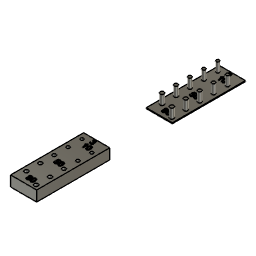
03 mm 3D Holes and Pins Kit v2 (Autodesk Fusion 360 design; units mm, degrees)
Autodesk Fusion 360 part; units mm, degrees
sketch "Schizzo1" plane through (0, 0, 0) normal (0, 0, 1) x (1, 0, 0)
  circle A0 centre (-272.0657, 86.4576) radius 1.5
  circle A1 centre (-256.0657, 66.4576) radius 1.65
  line L0 (-276.5657, 92.4576) -> (-251.5657, 92.4576)
  line L1 (-276.5657, 59.7909) -> (-251.5657, 59.7909) construction
  circle A2 centre (-272.0657, 73.1243) radius 1.6
  line L2 (-276.5657, 33.1243) -> (-251.5657, 33.1243) construction
  line L3 (-276.5657, 79.7909) -> (-251.5657, 79.7909) construction
  line L4 (-251.5657, 22.4576) -> (-276.5657, 22.4576)
  line L5 (-276.5657, 26.4576) -> (-251.5657, 26.4576) construction
  circle A3 centre (-256.0657, 39.7909) radius 1.85
  circle A4 centre (-272.0657, 33.1243) radius 1.9
  line L6 (-276.5657, 53.1243) -> (-251.5657, 53.1243) construction
  line L7 (-276.5657, 46.4576) -> (-251.5657, 46.4576) construction
  line L8 (-276.5657, 39.7909) -> (-251.5657, 39.7909) construction
  circle A5 centre (-256.0657, 26.4576) radius 1.95
  circle A6 centre (-272.0657, 46.4576) radius 1.8
  line L9 (-251.5657, 92.4576) -> (-251.5657, 22.4576)
  line L10 (-276.5657, 66.4576) -> (-251.5657, 66.4576) construction
  circle A7 centre (-256.0657, 53.1243) radius 1.75
  line L11 (-256.0657, 92.4576) -> (-256.0657, 22.4576) construction
  line L12 (-276.5657, 73.1243) -> (-251.5657, 73.1243) construction
  circle A8 centre (-272.0657, 59.7909) radius 1.7
  circle A9 centre (-256.0657, 79.7909) radius 1.55
  line L13 (-272.0657, 92.4576) -> (-272.0657, 22.4576) construction
  line L14 (-276.5657, 86.4576) -> (-251.5657, 86.4576) construction
  line L15 (-276.5657, 22.4576) -> (-276.5657, 92.4576)
  line L16 (-264.0657, 92.4576) -> (-264.0657, 22.4576) construction
  line L17 (-276.5657, -43.5424) -> (-251.5657, -43.5424) construction
  line L18 (-256.0657, -37.5424) -> (-256.0657, -107.5424) construction
  line L19 (-276.5657, -103.5424) -> (-251.5657, -103.5424) construction
  circle A10 centre (-256.0657, -103.5424) radius 1.95
  line L20 (-276.5657, -50.2091) -> (-251.5657, -50.2091) construction
  line L21 (-276.5657, -76.8757) -> (-251.5657, -76.8757) construction
  circle A11 centre (-272.0657, -56.8757) radius 1.6
  line L22 (-276.5657, -37.5424) -> (-251.5657, -37.5424)
  circle A12 centre (-256.0657, -76.8757) radius 1.75
  line L23 (-276.5657, -56.8757) -> (-251.5657, -56.8757) construction
  circle A13 centre (-256.0657, -63.5424) radius 1.65
  circle A14 centre (-256.0657, -50.2091) radius 1.55
  circle A15 centre (-272.0657, -70.2091) radius 1.7
  circle A16 centre (-272.0657, -43.5424) radius 1.5
  line L24 (-276.5657, -70.2091) -> (-251.5657, -70.2091) construction
  line L25 (-276.5657, -63.5424) -> (-251.5657, -63.5424) construction
  circle A17 centre (-272.0657, -83.5424) radius 1.8
  line L26 (-251.5657, -37.5424) -> (-251.5657, -107.5424)
  circle A18 centre (-272.0657, -96.8757) radius 1.9
  line L27 (-264.0657, -37.5424) -> (-264.0657, -107.5424) construction
  line L28 (-272.0657, -37.5424) -> (-272.0657, -107.5424) construction
  line L29 (-251.5657, -107.5424) -> (-276.5657, -107.5424)
  line L30 (-276.5657, -96.8757) -> (-251.5657, -96.8757) construction
  line L31 (-276.5657, -107.5424) -> (-276.5657, -37.5424)
  line L32 (-276.5657, -83.5424) -> (-251.5657, -83.5424) construction
  line L33 (-276.5657, -90.2091) -> (-251.5657, -90.2091) construction
  circle A19 centre (-256.0657, -90.2091) radius 1.85
  dimension "d172" = 5
  dimension "d173" = 5
  dimension "d174" = 5
  dimension "d175" = 5
  dimension "d178" = 60
  dimension "d179" = 0
  dimension "d180" = 25
  dimension "d181" = 70
  dimension "d182" = 8
  dimension "d183" = 6
  dimension "d184" = 3
  dimension "d185" = 3.2
  dimension "d186" = 3.1
  dimension "d187" = 3.4
  dimension "d188" = 3.6
  dimension "d189" = 3.8
  dimension "d190" = 3.3
  dimension "d191" = 3.5
  dimension "d192" = 3.7
  dimension "d193" = 3.9
  dimension "d194" = 5
  dimension "d195" = 5
  dimension "d196" = 5
  dimension "d197" = 5
  dimension "d200" = 60
  dimension "d201" = 0
  dimension "d202" = 25
  dimension "d203" = 70
  dimension "d204" = 8
  dimension "d205" = 6
  dimension "d206" = 3
  dimension "d207" = 3.2
  dimension "d208" = 3.1
  dimension "d209" = 3.4
  dimension "d210" = 3.6
  dimension "d211" = 3.8
  dimension "d212" = 3.3
  dimension "d213" = 3.5
  dimension "d214" = 3.7
  dimension "d215" = 3.9
  text T0 ".10" font "Arial" height 5 align centre spacing 1 along the path L3 letters at x, y, angle (-268.9207, 86.1143, 0) (-266.98, 86.1143, 0) (-263.0953, 86.1143, 0)
  text T1 ".90" font "Arial" height 5 align centre spacing 1 along the path L5 letters at x, y, angle (-268.9207, 32.7809, 0) (-266.98, 32.7809, 0) (-263.0953, 32.7809, 0)
  text T2 ".50" font "Arial" height 5 align centre spacing 1 along the path L6 letters at x, y, angle (-268.9207, 59.4476, 0) (-266.98, 59.4476, 0) (-263.0953, 59.4476, 0)
  text T3 "3" font "Arial" height 5 align centre spacing 1 along the path L14 letters at x, y, angle (-266.008, 92.7809, 0)
  text T4 "3" font "Arial" height 5 align centre spacing 1 along the path L17 letters at x, y, angle (-266.008, -37.2191, 0)
  text T5 ".90" font "Arial" height 5 align centre spacing 1 along the path L19 letters at x, y, angle (-268.9207, -97.2191, 0) (-266.98, -97.2191, 0) (-263.0953, -97.2191, 0)
  text T6 ".10" font "Arial" height 5 align centre spacing 1 along the path L20 letters at x, y, angle (-268.9207, -43.8857, 0) (-266.98, -43.8857, 0) (-263.0953, -43.8857, 0)
  text T7 ".50" font "Arial" height 5 align centre spacing 1 along the path L21 letters at x, y, angle (-268.9207, -70.5524, 0) (-266.98, -70.5524, 0) (-263.0953, -70.5524, 0)
  constraint horizontal L0
  constraint vertical L9
  constraint horizontal L4
  constraint vertical L15
  constraint coincident L13.start L0
  constraint coincident L13.end L4
  constraint perpendicular L4 L13
  constraint midpoint L16.start L0
  constraint perpendicular L0 L16
  constraint symmetric L13.start L11.start L16
  constraint symmetric L11.end L13.end L16
  constraint midpoint L16.end L4
  constraint coincident L14.start L15
  constraint coincident L14.end L9
  constraint perpendicular L9 L14
  constraint coincident A0.centre L13
  constraint coincident A0.centre L14
  constraint coincident A2.centre L12
  constraint coincident A2.centre L13
  constraint coincident A9.centre L3
  constraint coincident A9.centre L11
  constraint coincident A8.centre L13
  constraint coincident A8.centre L1
  constraint coincident A6.centre L13
  constraint coincident A6.centre L7
  constraint coincident A4.centre L2
  constraint coincident A4.centre L13
  constraint coincident A1.centre L10
  constraint coincident A1.centre L11
  constraint coincident A7.centre L11
  constraint coincident A7.centre L6
  constraint coincident A3.centre L8
  constraint coincident A3.centre L11
  constraint coincident A5.centre L5
  constraint coincident A5.centre L11
  constraint horizontal L22
  constraint vertical L26
  constraint horizontal L29
  constraint vertical L31
  constraint coincident L28.start L22
  constraint coincident L28.end L29
  constraint perpendicular L28 L29
  constraint midpoint L27.start L22
  constraint perpendicular L22 L27
  constraint symmetric L28.start L18.start L27
  constraint symmetric L18.end L28.end L27
  constraint midpoint L27.end L29
  constraint coincident L17.start L31
  constraint coincident L17.end L26
  constraint perpendicular L17 L26
  constraint coincident A16.centre L28
  constraint coincident A16.centre L17
  constraint coincident A11.centre L23
  constraint coincident A11.centre L28
  constraint coincident A14.centre L20
  constraint coincident A14.centre L18
  constraint coincident A15.centre L28
  constraint coincident A15.centre L24
  constraint coincident A17.centre L28
  constraint coincident A17.centre L32
  constraint coincident A18.centre L30
  constraint coincident A18.centre L28
  constraint coincident A13.centre L25
  constraint coincident A13.centre L18
  constraint coincident A12.centre L18
  constraint coincident A12.centre L21
  constraint coincident A19.centre L33
  constraint coincident A19.centre L18
  constraint coincident A10.centre L19
  constraint coincident A10.centre L18
  measures "d180" distance of L0.start L0.end
  measures "d181" distance of L4.end L0.start
  measures "d182" distance of L13 L16
  measures "d183" distance of L0 L14
  measures "d184" diameter of A0
  measures "d185" diameter of A2
  measures "d186" diameter of A9
  measures "d187" diameter of A8
  measures "d188" diameter of A6
  measures "d189" diameter of A4
  measures "d190" diameter of A1
  measures "d191" diameter of A7
  measures "d192" diameter of A3
  measures "d193" diameter of A5
  measures "d202" distance of L22.start L22.end
  measures "d203" distance of L29.end L22.start
  measures "d204" distance of L27 L28
  measures "d205" distance of L17 L22
  measures "d206" diameter of A16
  measures "d207" diameter of A11
  measures "d208" diameter of A14
  measures "d209" diameter of A15
  measures "d210" diameter of A17
  measures "d211" diameter of A18
  measures "d212" diameter of A13
  measures "d213" diameter of A12
  measures "d214" diameter of A19
  measures "d215" diameter of A10
extrude "Estrusione12" add sketch "Schizzo1" along normal blind 0.8 contours L0 L4 L9 L15 makes body 1
extrude "Estrusione13" add sketch "Schizzo1" along normal blind 10 contours A0 | A1 | A2 | A3 | A4 | A5 | A6 | A7 | A8 | A9 bodies 1
extrude "Estrusione14" add sketch "Schizzo1" along normal blind 0.4 from surface at 0.8 separate body text T3 T0 T2 T1 makes body 2 at (-267.8202, 26.6907, 0.8) makes body 3 at (-262.3711, 55.1522, 0.8) makes body 4 at (-265.1042, 57.8605, 0.8) makes body 5 at (-267.8202, 80.024, 0.8) makes body 6 at (-263.6654, 89.156, 0.8) makes body 7 at (-264.5824, 82.7684, 0.8) makes body 8 at (-262.3711, 81.8188, 0.8) makes body 9 at (-267.8202, 53.3573, 0.8) makes body 10 at (-263.6157, 28.7068, 0.8) makes body 11 at (-262.3711, 28.4855, 0.8)
extrude "Estrusione15" add sketch "Schizzo1" along normal blind 10 separate body contours L22 L26 L29 L31 makes body 12
extrude "Estrusione16" add sketch "Schizzo1" along normal blind 0.4 from surface at 10 separate body text T5 T7 T6 T4 makes body 13 at (-262.3711, -48.1812, 10) makes body 14 at (-264.5824, -47.2316, 10) makes body 15 at (-267.8202, -76.6427, 10) makes body 16 at (-262.3711, -101.5145, 10) makes body 17 at (-263.6157, -101.2932, 10) makes body 18 at (-267.8202, -103.3093, 10) makes body 19 at (-265.1042, -72.1395, 10) makes body 20 at (-262.3711, -74.8478, 10) makes body 21 at (-267.8202, -49.976, 10) makes body 22 at (-263.6654, -40.844, 10)
named bodies: "3 mm stud", "3 mm hole"
